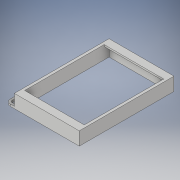
# Autodesk Inventor part: MiniBreadboardHolder
Saved by Autodesk Inventor 2018 (Build 220112000, 112)
## iProperties
Created: 2019-05-06
Part Number: MiniBreadboardHolder
Material: Generic
Document SubType Name: Modeling
Designer: jklei
Density: 1 g/cm^3
Appearance: Default
Author: jklei
Autodesk Inventor part; units mm, degrees
ref_plane "YZ Plane" through (0, 0, 0) normal (1, 0, 0) x (0, 1, 0)
ref_plane "XZ Plane" through (0, 0, 0) normal (0, 1, 0) x (-1, 0, 0)
ref_plane "XY Plane" through (0, 0, 0) normal (0, 0, 1) x (1, 0, 0)
sketch "Sketch1" plane through (0, 0, 0) normal (0, 1, 0) x (-1, 0, 0)
  line L0 (0, 0) -> (-57.15, 0)
  line L1 (-57.15, 0) -> (-57.15, -85.725)
  line L2 (-57.15, -85.725) -> (0, -85.725)
  line L3 (0, -85.725) -> (0, 0)
  line L4 (-59.69, -88.265) -> (-59.69, 2.54)
  line L5 (-59.69, 2.54) -> (2.54, 2.54)
  line L6 (2.54, 2.54) -> (2.54, -88.265)
  line L7 (2.54, -88.265) -> (-59.69, -88.265)
  dimension "d0" = 57.15
  dimension "d1" = 85.725
  dimension "d2" = 2.54
  constraints: 16 end point, 4 parallel, 2 perpendicular, 1 horizontal, 3 other
  measures "d0" distance of L2.end L1.end
  measures "d1" distance of L1.end L0.end
  measures "d2" distance between parallel lines of L1 L4
extrude "Extrusion1" add sketch "Sketch1" along normal blind 11.1125
sketch "Sketch2" plane through (0, 11.1125, 0) normal (0, 1, 0) x (1, 0, 0)
  line L0 (57.15, 0) -> (0, 0) projected
  line L1 (0, 85.725) -> (57.15, 85.725) projected
  line L2 (0, 0) -> (0, 85.725) projected
  line L3 (57.15, 85.725) -> (57.15, 0) projected
  line L4 (0, 85.725) -> (57.15, 85.725)
  line L5 (57.15, 85.725) -> (57.15, 80.9625)
  line L6 (57.15, 80.9625) -> (0, 80.9625)
  line L7 (0, 80.9625) -> (0, 85.725)
  line L8 (59.69, 88.265) -> (-2.54, 88.265) projected
  line L9 (-2.54, -2.54) -> (59.69, -2.54) projected
  line L10 (0, 0) -> (57.15, 0)
  line L11 (57.15, 0) -> (57.15, 4.7625)
  line L12 (57.15, 4.7625) -> (0, 4.7625)
  line L13 (0, 4.7625) -> (0, 0)
  line L14 (0, 0) -> (0, 85.725) projected
  line L15 (0, 85.725) -> (57.15, 85.725) projected
  line L16 (57.15, 85.725) -> (57.15, 0) projected
  line L17 (57.15, 0) -> (0, 0) projected
  line L18 (59.69, -2.54) -> (59.69, 88.265) projected
  line L19 (59.69, 88.265) -> (-2.54, 88.265) projected
  line L20 (-2.54, 88.265) -> (-2.54, -2.54) projected
  line L21 (-2.54, -2.54) -> (59.69, -2.54) projected
  dimension "d5" = 4.7625
  dimension "d6" = 4.7625
  constraints: 16 end point, 4 parallel, 2 horizontal, 2 perpendicular, 2 point on line
  measures "d5" distance of L4.end L5.end
  measures "d6" distance of L11.end L10.end
extrude "Extrusion2" add sketch "Sketch2" along normal blind 1.5875 contours L0 L2 L12 L3 | L6 L2 L1 L3 | L18 L9 L20 L8
sketch "Sketch4" plane through (-2.54, 0, -88.265) normal (-1, 0, 0) x (0, 0, 1)
  line L0 (90.805, 0) -> (0, 0) projected
  line L1 (90.805, 0) -> (90.805, 12.7) projected
  line L2 (0, 12.7) -> (90.805, 12.7) projected
  line L3 (0, 0) -> (0, 12.7) projected
  line L4 (90.805, 0) -> (90.805, 12.7) projected
  line L5 (90.805, 0) -> (27.305, 0)
  line L6 (27.305, 0) -> (27.305, 2)
  line L7 (27.305, 2) -> (90.805, 2)
  line L8 (90.805, 2) -> (90.805, 0)
  point P0 (88.265, 0)
  dimension "d13" = 63.5
  dimension "d14" = 2
  constraints: 8 end point, 2 parallel, 1 horizontal, 1 perpendicular
  measures "d13" distance of L6.end L7.end
  measures "d14" distance of L5.end L6.end
extrude "Extrusion4" add sketch "Sketch4" along normal blind 8 contours L0 L6 L7 L1
fillet "Fillet2" radius 4 2 edges at (-10.54, 1, 2.54) (-10.54, 1, -60.96)
sketch "Sketch5" plane through (-2.54, 2, 2.54) normal (0, 1, 0) x (1, 0, 0)
  line L0 (-8, 4) -> (-8, 59.5) projected
  line L1 (-8, 4) -> (0, 4)
  line L2 (0, 63.5) -> (0, 0) projected
  circle A0 centre (-4, 4) radius 2.1
  line L3 (-8, 59.5) -> (0, 59.5)
  circle A1 centre (-4, 59.5) radius 2.1
  point P0 (2.54, 2.54)
  dimension "d20" = 4.2
  dimension "d21" = 4.2
  constraints: 4 end point, 2 centre point, 2 midpoint, 2 point on line, 1 horizontal, 1 perpendicular
  measures "d20" diameter of A0
  measures "d21" diameter of A1
extrude "Extrusion5" cut sketch "Sketch5" against normal up to next contours A0 L1 | L1 A0 | A1 L3 | L3 A1
body "Solid1"
